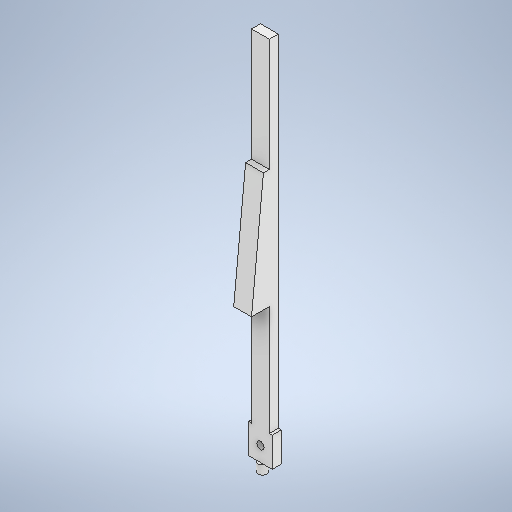
# Autodesk Inventor part: SchubstangeA
Saved by Autodesk Inventor 2025 (Build 290162010, 162A)
## iProperties
Created: 2024-11-26
Part Number: SchubstangeA
Material: PC/ABS-Kunststoff, 3DDruck, PLA
Document SubType Name: Modeling
Designer: Admin
Density: 1.1 g/cm^3
Appearance: Glatt - Weiß(2)
Author: Admin
Autodesk Inventor part; units mm, degrees
ref_plane "YZ Plane" through (0, 0, 0) normal (1, 0, 0) x (0, 1, 0)
ref_plane "XZ Plane" through (0, 0, 0) normal (0, 1, 0) x (-1, 0, 0)
ref_plane "XY Plane" through (0, 0, 0) normal (0, 0, 1) x (1, 0, 0)
sketch "Skizze1" plane through (0, 0, 0) normal (0, 1, 0) x (-1, 0, 0)
  line L0 (6.8592, -116.2444) -> (0.8592, -116.2444)
  line L1 (0.8592, -116.2444) -> (0.8592, 8.7556)
  line L2 (6.8592, 8.7556) -> (6.8592, -116.2444)
  line L3 (7.8592, -116.2444) -> (-0.1408, -116.2444)
  line L4 (-0.1408, -116.2444) -> (-0.1408, -106.2444)
  line L5 (-0.1408, -106.2444) -> (7.8592, -106.2444)
  line L6 (7.8592, -106.2444) -> (7.8592, -116.2444)
  line L7 (3.8592, 157.3916) -> (3.8592, -262.6084)
  line L8 (6.8592, 8.7556) -> (0.8592, 8.7556)
  point P0 (0, 0)
  point P1 (0.8592, -106.2444)
  point P2 (6.8592, -106.2444)
  point P3 (6.8592, -116.2444)
  point P4 (3.8592, -116.2444)
  dimension "d1" = 125
  dimension "d9" = 6
  dimension "d25" = 8
  dimension "d26" = 10
  dimension "d27" = 1
  constraints: 18 end point, 4 horizontal, 3 parallel, 2 perpendicular, 1 collinear, 1 midpoint, 1 point on line, 1 vertical, 2 other
  measures "d1" distance of L0.end L1.end
  measures "d9" distance of L0.start L0.end
  measures "d25" distance of L4.end L5.end
  measures "d26" distance of L3.end L4.end
  measures "d27" distance of L3.end L0.end
extrude "Extrusion1" add sketch "Skizze1" along normal blind 3
sketch "Skizze2" plane through (0, 3, 0) normal (0, 1, 0) x (1, 0, 0)
  line L0 (-3.8592, 111.2444) -> (-6.8592, 111.2444) construction
  line L1 (-3.8592, 111.2444) -> (-0.8592, 111.2444) construction
  line L2 (-0.8592, -8.7556) -> (-0.8592, 106.2444) construction
  line L3 (-6.8592, 106.2444) -> (-6.8592, -8.7556) construction
  line L4 (0.1408, 116.2444) -> (-7.8592, 116.2444) projected
  point P0 (0, 0)
  point P1 (-0.8592, 16.2444)
  point P2 (-6.8592, 16.2444)
  dimension "d28" = 5
  constraints: 4 end point, 2 horizontal, 2 point on line, 1 collinear
  measures "d28" distance from line of L4 L0.start
hole "Bohrung1" at (-3.8592, 3, -111.2444) direction (0, -1, 0) diameter 2.459 end through all thread size "M3x0.5" class "6H" standard "ANSI Metric M Profile"
sketch "Skizze3" plane through (0.1408, 0, -116.2444) normal (0, 0, -1) x (-1, 0, 0)
  line L0 (4, 0) -> (4, 0.7)
  circle A0 centre (4, 0.7) radius 1.5
  line L1 (0, 0) -> (8, 0) projected
  point P0 (0.1408, 0)
  dimension "d29" = 3
  dimension "d30" = 0.7
  constraints: 3 end point, 1 centre point, 1 midpoint, 1 perpendicular
  measures "d29" diameter of A0
  measures "d30" distance from line of L1 L0.end
extrude "Extrusion2" add sketch "Skizze3" along normal blind 3
sketch "Skizze4" plane through (0, 0, 0) normal (0, -1, 0) x (1, 0, 0)
  line L0 (-0.8592, 8.7556) -> (-0.8592, -106.2444) projected
  line L1 (-6.8592, -69.2444) -> (-0.8592, -69.2444)
  line L2 (-0.8592, -69.2444) -> (-0.8592, -29.2444)
  line L3 (-0.8592, -29.2444) -> (-6.8592, -29.2444)
  line L4 (-6.8592, -29.2444) -> (-6.8592, -69.2444)
  point P0 (0, 0)
  point P1 (-0.8592, -69.2444)
  point P2 (-6.8592, -106.2444)
  dimension "d34" = 40
  dimension "d37" = 37
  dimension "d38" = 6
  constraints: 8 end point, 2 parallel, 1 horizontal, 1 perpendicular, 1 point on line
  measures "d34" distance of L2.end L1.end
  measures "d37" distance from line of point (-6.859, -106.244) L1
  measures "d38" distance of L1.start L1.end
extrude "Extrusion3" add sketch "Skizze4" along normal blind 6
chamfer "Fasen1" distance 40 distance2 4 1 edges at (-3.8592, -6, -29.2444) measured on face at (-4.8592, -6, -42.5778)
